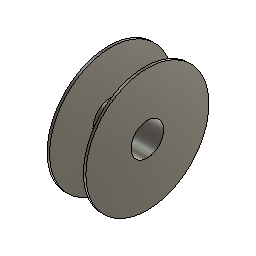
Filament Spool (Autodesk Fusion 360 design; units mm, degrees)
Autodesk Fusion 360 part; units mm, degrees
sketch "Sketch1" plane through (0, 0, 0) normal (1, 0, 0) x (0, 1, 0)
  circle A0 centre (0, 0) radius 100
  dimension "d1" = 200
  constraint coincident A0.centre origin
  measures "d1" diameter of A0
extrude "Extrude1" add sketch "Sketch1" along normal blind 4
sketch "Sketch2" plane through (4, 0, 0) normal (1, 0, 0) x (0, 1, 0)
  circle A0 centre (0, 0) radius 100
  circle A1 centre (0, 0) radius 26.5
  circle A2 centre (0, 0) radius 29.5
  dimension "d4" = 53
  dimension "d5" = 3
  constraint concentric A0 A1
  measures "d4" diameter of A1
extrude "Extrude2" add sketch "Sketch2" along normal blind 27.5 contours A2
extrude "Extrude3" cut 1 faces at (4, -6.4753, 6.0082) along direction (-1, 0, 0) blind 40
mirror "Mirror1" about plane through (31.5, 0, 0) normal (1, 0, 0) of bodies 1 merged
